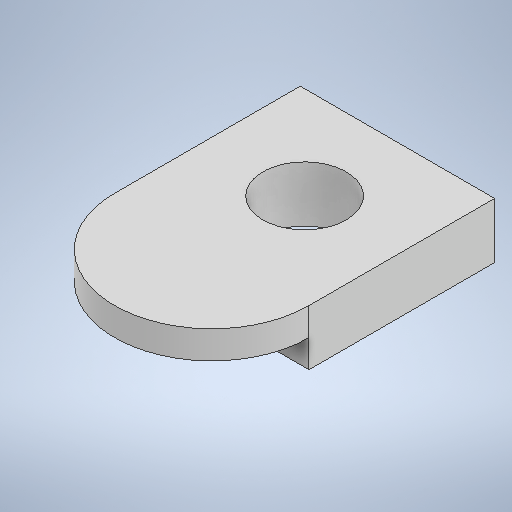
# Autodesk Inventor part: sunfoundernub
Saved by Autodesk Inventor 2025 (Build 290162000, 162)
## iProperties
Created: 2025-05-31
Part Number: sunfoundernub
Material: Generic
Document SubType Name: Modeling
Designer: ethan
Density: 1 g/cm^3
Appearance: Default
Author: ethan
Autodesk Inventor part; units mm, degrees
ref_plane "YZ Plane" through (0, 0, 0) normal (1, 0, 0) x (0, 1, 0)
ref_plane "XZ Plane" through (0, 0, 0) normal (0, 1, 0) x (-1, 0, 0)
ref_plane "XY Plane" through (0, 0, 0) normal (0, 0, 1) x (1, 0, 0)
sketch "Sketch1" plane through (0, 0, 0) normal (0, 1, 0) x (-1, 0, 0)
  line L0 (0, 0) -> (7, 0)
  line L1 (7, 0) -> (7, -6.684)
  line L2 (7, -6.684) -> (0, -6.684)
  line L3 (0, -6.684) -> (0, 0)
  line L4 (3.5, -6.684) -> (3.5, -3.342)
  circle A0 centre (3.5, -3.342) radius 1.5
  dimension "d0" = 7
  dimension "d1" = 6.684
  dimension "d2" = 3.342
  dimension "d3" = 3
  constraints: 10 end point, 2 parallel, 1 centre point, 1 coincident, 1 horizontal, 1 midpoint, 1 perpendicular, 1 vertical
  measures "d0" distance of L1.end L2.end
  measures "d1" distance of L0.end L1.end
  measures "d2" distance of L4.start L4.end
  measures "d3" diameter of A0
extrude "Extrusion1" add sketch "Sketch1" along normal blind 1
sketch "Sketch2" plane through (0, 1, 0) normal (0, 1, 0) x (1, 0, 0)
  line L0 (-7, 6.684) -> (-7, 0) projected
  line L1 (-7, 0) -> (0, 0) projected
  line L2 (0, 0) -> (0, 6.684) projected
  line L3 (0, 6.684) -> (-7, 6.684) projected
  circle A0 centre (-3.5, 3.342) radius 1.5 projected
  arc A1 (-7, 0) -> (0, 0) centre (-3.5, 0) ccw
  constraints: 2 point on circle, 2 tangent, 1 centre point
extrude "Extrusion2" add sketch "Sketch2" along normal blind 1
body "Solid1"
